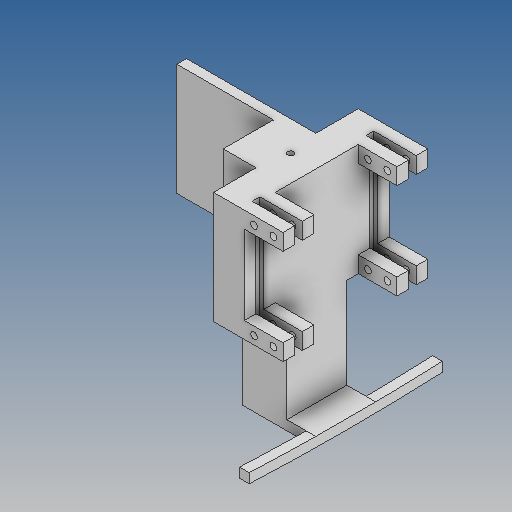
# Autodesk Inventor part: Korpus
Saved by Autodesk Inventor 2026.2 (Build 302298000, 298)
## iProperties
Created: 2025-08-31
Part Number: Korpus
Material: Generisch
Document SubType Name: Modeling
Designer: weyer
Density: 1 g/cm^3
Appearance: Vorgabe
Author: weyer
Autodesk Inventor part; units mm, degrees
ref_plane "YZ Plane" through (0, 0, 0) normal (1, 0, 0) x (0, 1, 0)
ref_plane "XZ Plane" through (0, 0, 0) normal (0, 1, 0) x (-1, 0, 0)
ref_plane "XY Plane" through (0, 0, 0) normal (0, 0, 1) x (1, 0, 0)
sketch "Skizze1" plane through (0, 0, 0) normal (0, 0, 1) x (1, 0, 0)
  line L0 (-9.5, -10.5) -> (7.5, -10.5)
  line L1 (7.5, -10.5) -> (7.5, 10.5)
  line L2 (7.5, 10.5) -> (-9.5, 10.5)
  line L3 (-14.1, 0) -> (18.1, 0) projected
  line L4 (0, -21.7) -> (0, 21.7) projected
  line L5 (-9.5, -10.5) -> (-9.5, -15.5)
  line L6 (-9.5, -15.5) -> (13.5, -15.5)
  line L7 (-9.5, 10.5) -> (-9.5, 15.5)
  line L8 (-9.5, 15.5) -> (13.5, 15.5)
  line L9 (13.5, 15.5) -> (13.5, -15.5)
  point P0 (0, 0)
  dimension "d2" = 21
  dimension "d4" = 7.5
  dimension "d5" = 5
  dimension "d8" = 5
  dimension "d9" = 23
  dimension "d147" = 6
  dimension "d148" = 23
  constraints: 16 end point, 4 perpendicular, 2 vertical, 1 horizontal, 1 other
  measures "d2" distance between parallel lines of L0 L2
  measures "d4" distance between parallel lines of L1 L4
  measures "d5" distance of L0.start L5.end
  measures "d8" distance of L2.end L7.end
  measures "d9" distance of L7.end L8.end
  measures "d147" distance between parallel lines of L1 L9
  measures "d148" distance between parallel lines of L9 L5
extrude "Tower" add sketch "Skizze1" against normal blind 100 contours L0 L4 L6 L5 | L0 L1 L3 L9 L6 L4 | L1 L2 L4 L8 L9 L3 | L2 L7 L8 L4
ref_plane "Arbeitsebene1" through (0, 0, -100) normal (0, 0, -1) x (-1, 0, 0)
sketch "Skizze6" plane through (-9.5, 15.5, 0) normal (0, 1, 0) x (1, 0, 0)
  line L0 (23, 0) -> (23, 100) projected
  line L1 (23, 66.4131) -> (23, 0)
  line L2 (246, -7) -> (246, -5)
  line L3 (0, 0) -> (0, 100) projected
  line L4 (0, 0) -> (23, 0) projected
  line L5 (0, 0) -> (0, 100) projected
  line L6 (23, 100) -> (0, 100) projected
  line L7 (23, 0) -> (23, 100) projected
  line L8 (0, 0) -> (23, 0)
  line L9 (23, 0) -> (23, -10)
  line L10 (23, -10) -> (0, -10)
  line L11 (0, -10) -> (0, 0)
  dimension "d199" = 10
  constraints: 12 end point, 2 parallel, 1 horizontal, 1 perpendicular, 1 point on line, 1 vertical
  measures "d199" distance of L8.end L9.end
extrude "Gripperbogen" add sketch "Skizze6" against normal blind 31 contours L9 L10 L11 L4
sketch "Skizze12" plane through (0, 0, -100) normal (0, 0, -1) x (-1, 0, 0)
  line L0 (-214.5, 9.5) -> (-236.5, 9.5) projected
  line L1 (-236.5, 15.5) -> (-236.5, 9.5) projected
  line L2 (9.5, 15.5) -> (-236.5, 15.5) projected
  line L3 (9.5, 15.5) -> (9.5, -15.5) projected
  line L4 (-136.5, -15.5) -> (9.5, -15.5) projected
  line L5 (-136.5, -15.5) -> (-206.5, 0) projected
  line L6 (-206.5, 0) -> (-236.5, 0) projected
  line L7 (-236.5, 6) -> (-236.5, 0) projected
  line L8 (-236.5, 6) -> (-214.5, 6) projected
  line L9 (-214.5, 6) -> (-214.5, 9.5) projected
  line L10 (-7.5, 10.5) -> (9.5, 10.5) projected
  line L11 (9.5, 10.5) -> (9.5, 15.5) projected
  line L12 (9.5, 15.5) -> (-13.5, 15.5) projected
  line L13 (-13.5, 15.5) -> (-13.5, -15.5) projected
  line L14 (-13.5, -15.5) -> (9.5, -15.5) projected
  line L15 (9.5, -15.5) -> (9.5, -10.5) projected
  line L16 (9.5, -10.5) -> (-7.5, -10.5) projected
  line L17 (-7.5, -10.5) -> (-7.5, 10.5) projected
  line L18 (-13.5, 15.5) -> (-13.5, -15.5) projected
  line L19 (-13.5, -15.5) -> (9.5, -15.5)
  line L20 (9.5, -15.5) -> (9.5, 15.5)
  line L21 (9.5, 15.5) -> (-13.5, 15.5)
  line L22 (-13.5, 15.5) -> (-13.5, -15.5)
  point P0 (9.5, 25.25)
  point P1 (-13.5, -5.25)
  point P2 (-13.5, 15.5)
  constraints: 8 end point, 2 parallel, 1 horizontal, 1 perpendicular
extrude "Extrusion10" add sketch "Skizze12" against normal blind 10 contours L2 L3 L10 L17 L16 L4 L13 | L3 L16 L17 L10
ref_plane "Arbeitsebene3" through (0, 0, -113.5) normal (0, 0, -1) x (-1, 0, 0)
ref_plane "Arbeitsebene4" through (-9.5, -5.25, -113.5) normal (-1, 0, 0) x (0, 0, 1)
sketch "Skizze18" plane through (0, 0, -90) normal (0, 0, 1) x (1, 0, 0)
  line L0 (7.5, 10.5) -> (7.5, -10.5) projected
  line L1 (-9.5, 10.5) -> (7.5, 10.5) projected
  circle A0 centre (2, 0) radius 2.75
  line L2 (7.5, -10.5) -> (-9.5, -10.5) projected
  line L3 (-9.5, 10.5) -> (-9.5, -10.5) projected
  point P0 (0, 0)
  dimension "d132" = 5.5
  dimension "d154" = 0
  dimension "d155" = 11.5
  dimension "d161" = 21
  dimension "d162" = 17
  constraints: 1 centre point
  measures "d132" diameter of A0
  measures "d154" vertical distance of point (0, 0) A0.centre
  measures "d155" distance from line of L3 A0.centre
  measures "d161" distance between parallel lines of L2 L1
  measures "d162" distance between parallel lines of L0 L3
extrude "Extrusion15" cut sketch "Skizze18" against normal through all contours A0
sketch "Skizze19" plane through (-9.5, -15.5, -100) normal (-1, 0, 0) x (0, 0, 1)
  line L0 (0, 0) -> (0, 31) projected
  line L1 (100, 26) -> (10, 26) projected
  line L2 (100, 5) -> (10, 5) projected
  line L3 (30, 31) -> (30, 0)
  line L4 (10, 26) -> (10, 5) projected
  line L5 (10, 26) -> (0, 26)
  line L6 (10, 5) -> (0, 5)
  line L7 (100, 26) -> (110, 26)
  line L8 (10, 26) -> (10, 5) projected
  line L9 (110, 0) -> (0, 0) projected
  line L10 (110, 31) -> (110, 0) projected
  line L11 (0, 31) -> (110, 31) projected
  line L12 (100, 26) -> (100, 5) projected
  point P0 (100, 15.5)
  point P1 (23.5, 25.5)
  point P2 (23.5, 5)
  point P3 (30, 26)
  point P4 (30, 5)
  point P5 (20, 10.25)
  point P6 (30, 0)
  dimension "d201" = 80
  constraints: 8 end point, 2 perpendicular, 2 point on line, 1 other
  measures "d201" distance between parallel lines of L3 L10
extrude "Extrusion16" add sketch "Skizze19" along normal blind 10 contours L3 L2 L12 L7 L10 L9 | L3 L11 L10 L7 L1
sketch "Skizze15" plane through (-9.5, -15.5, -100) normal (0, -1, 0) x (1, 0, 0)
  line L0 (23, 0) -> (0, 0) projected
  circle A0 centre (-1, 49) radius 2.25
  circle A1 centre (-1, 89) radius 2.25
  line L1 (23, 0) -> (23, 110) projected
  line L2 (23, 110) -> (-10, 110) projected
  line L3 (0, 30) -> (0, 0) projected
  line L4 (-10, 30) -> (-10, 110) projected
  line L5 (0, 30) -> (-10, 30) projected
  point P0 (9.5, 100)
  dimension "d138" = 4.5
  dimension "d142" = 4.5
  dimension "d143" = 40
  dimension "d200" = 24
  constraints: 2 centre point, 1 vertical alignment
  measures "d138" diameter of A0
  measures "d142" diameter of A1
  measures "d143" distance of A1.centre A0.centre
  measures "d200" distance from line of L1 A1.centre
extrude "Extrusion13" cut sketch "Skizze15" against normal blind 100 contours A0 | A1
sketch "Skizze35" plane through (13.5, -15.5, -100) normal (1, 0, 0) x (0, 0, -1)
  line L0 (-100, 31) -> (0, 31) projected
  line L1 (-100, 0) -> (0, 0) projected
  line L2 (0, 31) -> (0, 0) projected
  line L3 (0, 31) -> (0, 0) projected
  line L4 (0, 0) -> (-5, 0)
  line L5 (-5, 0) -> (-5, 31)
  line L6 (-5, 31) -> (0, 31)
  line L7 (0, 31) -> (0, 0)
  line L8 (-110, 31) -> (0, 31) projected
  line L9 (-110, 31) -> (-110, 0) projected
  line L10 (0, 0) -> (-110, 0) projected
  point P0 (-29.8382, 31)
  point P1 (-29.8382, 0)
  point P2 (-100, 15.5)
  point P3 (-5, 31)
  point P4 (-5, 0)
  point P5 (-80, 31)
  point P6 (-80, 0)
  dimension "d176" = 5
  constraints: 8 end point, 2 parallel, 1 horizontal, 1 perpendicular
  measures "d176" distance of L5.end L6.end
extrude "Extrusion22" add sketch "Skizze35" along normal blind 10 contours L0 L2 L1 L5
sketch "Skizze36" plane through (23.5, -15.5, -100) normal (1, 0, 0) x (0, 0, -1)
  line L0 (-5, 0) -> (0, 0) projected
  line L1 (0, 0) -> (0, 31) projected
  line L2 (0, 31) -> (-5, 31) projected
  line L3 (-5, 31) -> (-5, 0) projected
  arc A0 (-9.879, -89.9986) -> (-9.879, 121.0014) centre (-1120.404, 15.5014) ccw
  line L4 (-5, 15.5) -> (0, 15.5)
  arc A1 (-4.9014, -90.4715) -> (-4.9014, 121.4742) centre (-1120.404, 15.5014) ccw
  line L5 (-5, 15.5) -> (0, 15.5)
  line L6 (-14.7679, -34.5) -> (17.3967, -34.5)
  line L7 (-14.7679, 65.5) -> (14.0644, 65.5)
  point P0 (-100, 15.5)
  point P1 (-0.9951, 65.5)
  point P2 (-6.0001, 65.5)
  point P3 (-4.9867, 31)
  point P4 (-4.9867, 0)
  point P5 (-6.0002, -34.5)
  point P6 (-0.9952, -34.5)
  dimension "d181" = 5
  dimension "d182" = 100
  constraints: 8 end point, 4 point on circle, 3 horizontal, 2 centre point, 2 midpoint, 1 other
  measures "d181" radial gap between concentric circles of A0 A1
  measures "d182" distance between parallel lines of L7 L6
extrude "Extrusion23" add sketch "Skizze36" along normal blind 5
sketch "Skizze40" plane through (-19.5, -15.5, 10) normal (0, -1, 0) x (1, 0, 0)
  line L0 (33, -105) -> (33, 0) projected
  line L1 (33, 0) -> (0, 0) projected
  line L2 (33, 0) -> (17, 0)
  line L3 (17, 0) -> (17, -58)
  line L4 (17, -58) -> (33, -58)
  line L5 (33, -58) -> (33, 0)
  point P0 (19.5, -10)
  point P1 (17, 0)
  dimension "d202" = 16
  dimension "d203" = 58
  constraints: 8 end point, 2 parallel, 1 horizontal, 1 perpendicular
  measures "d202" distance of L4.end L3.end
  measures "d203" distance of L3.end L2.end
extrude "Extrusion26" add sketch "Skizze40" along normal blind 22
sketch "Skizze41" plane through (-19.5, 15.5, 10) normal (0, 1, 0) x (1, 0, 0)
  line L0 (0, 0) -> (33, 0) projected
  line L1 (33, 0) -> (33, 105) projected
  line L2 (33, 58) -> (33, 0) projected
  line L3 (33, 0) -> (17, 0) projected
  line L4 (17, 0) -> (17, 58) projected
  line L5 (17, 58) -> (33, 58) projected
  point P0 (19.5, 10)
extrude "Extrusion27" add sketch "Skizze41" along normal blind 22
sketch "Skizze42" plane through (13.5, -15.5, -95) normal (1, 0, 0) x (0, 0, -1)
  line L0 (0, 0) -> (0, 31) projected
  line L1 (-47, 31) -> (-47, 53) projected
  line L2 (-105, -22) -> (-105, 53) projected
  line L3 (-47, 0) -> (-47, -22) projected
  line L4 (-47, 43) -> (-105, 43)
  line L5 (-105, 43) -> (-105, 47)
  line L6 (-105, 47) -> (-47, 47)
  line L7 (-47, 47) -> (-47, 43)
  line L8 (-47, -12) -> (-105, -12)
  line L9 (-105, -12) -> (-105, -16)
  line L10 (-105, -16) -> (-47, -16)
  line L11 (-47, -16) -> (-47, -12)
  line L12 (-105, 15.5) -> (0, 15.5)
  line L13 (-105, 53) -> (-47, 53) projected
  line L14 (-47, -22) -> (-105, -22) projected
  point P0 (-95, 15.5)
  point P1 (-105, 43)
  dimension "d208" = 4
  dimension "d209" = 4
  dimension "d214" = 6
  dimension "d215" = 6
  constraints: 18 end point, 4 parallel, 4 point on line, 2 horizontal, 2 midpoint, 2 perpendicular, 1 other
  measures "d208" distance between parallel lines of L6 L4
  measures "d209" distance between parallel lines of L10 L8
  measures "d214" distance between parallel lines of L13 L6
  measures "d215" distance between parallel lines of L14 L10
extrude "Extrusion28" cut sketch "Skizze42" against normal blind 2 contours L4 L2 L6 L1 | L2 L8 L3 L10
sketch "Skizze44" plane through (13.5, -15.5, -95) normal (1, 0, 0) x (0, 0, -1)
  line L0 (-47, 43) -> (-105, 43) projected
  line L1 (-105, -12) -> (-105, 43) projected
  line L2 (-105, -12) -> (-47, -12) projected
  line L3 (-47, 0) -> (-47, -12) projected
  line L4 (-47, 31) -> (-47, 43) projected
  line L5 (-47, -16) -> (-105, -16) projected
  line L6 (-105, -22) -> (-105, -16) projected
  line L7 (-47, -22) -> (-105, -22) projected
  line L8 (-47, -16) -> (-47, -22) projected
  line L9 (-105, 47) -> (-47, 47) projected
  line L10 (-47, 47) -> (-47, 53) projected
  line L11 (-105, 53) -> (-47, 53) projected
  line L12 (-105, 47) -> (-105, 53) projected
  line L13 (-105, -22) -> (-96.5, -22)
  line L14 (-96.5, -22) -> (-96.5, -16)
  line L15 (-96.5, -16) -> (-105, -16)
  line L16 (-105, -16) -> (-105, -22)
  line L17 (-55.5, -22) -> (-47, -22)
  line L18 (-47, -22) -> (-47, -16)
  line L19 (-47, -16) -> (-55.5, -16)
  line L20 (-55.5, -16) -> (-55.5, -22)
  line L21 (-47, -12) -> (-55.5, -12)
  line L22 (-55.5, -12) -> (-55.5, -6)
  line L23 (-55.5, -6) -> (-47, -6)
  line L24 (-47, -6) -> (-47, -12)
  line L25 (-105, -12) -> (-96.5, -12)
  line L26 (-96.5, -12) -> (-96.5, -6)
  line L27 (-96.5, -6) -> (-105, -6)
  line L28 (-105, -6) -> (-105, -12)
  line L29 (-105, 37) -> (-96.5, 37)
  line L30 (-96.5, 37) -> (-96.5, 49)
  line L31 (-96.5, 49) -> (-100.5, 49)
  line L32 (-55.5, 53) -> (-55.5, 59)
  line L33 (-96.5, 53) -> (-94.5, 53)
  line L34 (-96.5, 47) -> (-96.5, 53)
  line L35 (-55.5, 37) -> (-47, 37)
  line L36 (-55.5, 53) -> (-55.5, 47)
  line L37 (-55.5, 43) -> (-55.5, 37)
  point P0 (-95, 15.5)
  point P1 (-55.5, -19)
  point P2 (-55.5, -9)
  point P3 (-96.5, -19)
  point P4 (-96.5, -9)
  point P5 (-51.25, -6)
  point P6 (-100.75, -6)
  point P7 (-55.5, 56)
  point P8 (-96.5, 43)
  point P9 (-46.25, 53)
  point P10 (-95.5, 53)
  point P11 (-105, 50)
  point P12 (-76, 53)
  point P13 (-48.75, 37)
  point P14 (-98, 37)
  point P15 (-96.5, 50)
  point P16 (-55.5, 53)
  point P17 (-55.5, 50)
  point P18 (-100, 40)
  point P19 (-96.5, 43)
  point P20 (-47, -6)
  point P21 (-55.5, -12)
  point P22 (-96.5, -12)
  point P23 (-51.25, 37)
  point P24 (-100.75, 37)
  point P25 (-55.5, 40)
  dimension "d216" = 8.5
  dimension "d217" = 8.5
  dimension "d218" = 41
  dimension "d219" = 6
  dimension "d223" = 6
  dimension "d224" = 6
  constraints: 50 end point, 16 midpoint, 9 parallel, 9 point on line, 9 vertical alignment, 6 horizontal alignment, 6 perpendicular, 5 horizontal, 3 vertical
  measures "d216" distance of L15.end L14.end
  measures "d217" distance of L19.end L18.end
  measures "d218" distance between parallel lines of L20 L14
  measures "d219" distance of L21.end L22.end
  measures "d223" distance of L32.start L32.end
  measures "d224" distance between parallel lines of L0 L29
extrude "Extrusion29" add sketch "Skizze44" along normal blind 20 contours L4 L35 L37 L0 | L30 L29 L1 L0 | L1 L27 L26 L2 | L22 L23 L3 L2 | L8 L7 L20 L5 | L14 L7 L6 L5 | L12 L11 L34 L30 L9 | L36 L11 L10 L9
sketch "Skizze45" plane through (-19.5, -37.5, 10) normal (0, -1, 0) x (1, 0, 0)
  line L0 (53, 0) -> (53, -8.5) projected
  line L1 (17, 0) -> (17, -58) projected
  line L2 (53, -49.5) -> (53, -58) projected
  line L3 (33, -58) -> (33, -49.5) projected
  line L4 (53, -4.25) -> (17, -4.25)
  line L5 (53, -53.75) -> (17, -53.75)
  circle A0 centre (38, -53.75) radius 1.75
  circle A1 centre (48, -53.75) radius 1.75
  circle A2 centre (38, -4.25) radius 1.75
  circle A3 centre (48, -4.25) radius 1.75
  line L6 (33, -49.5) -> (33, -8.5) projected
  point P0 (19.5, -10)
  dimension "d227" = 3.5
  dimension "d228" = 3.5
  dimension "d229" = 3.5
  dimension "d230" = 3.5
  dimension "d231" = 5
  dimension "d237" = 5
  constraints: 6 point on line, 4 centre point, 4 end point, 2 midpoint, 2 perpendicular, 2 vertical alignment
  measures "d227" diameter of A0
  measures "d228" diameter of A1
  measures "d229" diameter of A2
  measures "d230" diameter of A3
  measures "d231" distance from line of L0 A3.centre
  measures "d237" distance from line of L6 A2.centre
extrude "Extrusion30" cut sketch "Skizze45" against normal blind 100
sketch "Skizze46" plane through (-19.5, -15.5, -100) normal (-1, 0, 0) x (0, 0, 1)
  line L0 (30, 26) -> (100, 26) projected
  line L1 (110, 0) -> (110, 31) projected
  line L2 (110, 31) -> (30, 31) projected
  line L3 (52, 31) -> (52, 53) projected
  line L4 (110, -22) -> (52, -22) projected
  line L5 (52, 53) -> (52, -22)
  line L6 (100, 26) -> (110, 26)
  point P0 (100, 15.5)
  point P1 (52, 26)
  constraints: 4 end point, 2 perpendicular, 1 point on line
extrude "Extrusion31" add sketch "Skizze46" along normal blind 50
sketch "Skizze47" plane through (-19.5, -15.5, 10) normal (0, 0, 1) x (1, 0, 0)
  circle A0 centre (21.5, 15.5) radius 2.75 projected
  line L0 (27, 5) -> (10, 5) projected
  line L1 (27, 26) -> (27, 5) projected
  line L2 (10, 26) -> (27, 26) projected
  line L3 (10, 26) -> (10, 5) projected
  circle A1 centre (19.5, 15.5) radius 1.6
  dimension "d238" = 3.2
  constraints: 1 centre point, 1 coincident
  measures "d238" diameter of A1
extrude "Extrusion32" cut sketch "Skizze47" against normal blind 10 contours A1 A0 | A0 A1 picked at (19.5471, 15.5) picked at (18.4804, 15.5)
